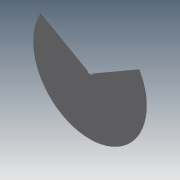
# Autodesk Inventor part: view2
Saved by Autodesk Inventor 2011 (Build 150239000, 239)
## iProperties
Created: 2011-12-04
Part Number: view2
Document SubType Name: Modeling
Designer: Matthew
Density: 1 g/cm^3
Author: Matthew
Autodesk Inventor part; units mm, degrees
ref_plane "YZ Plane" through (0, 0, 0) normal (1, 0, 0) x (0, 1, 0)
ref_plane "XZ Plane" through (0, 0, 0) normal (0, 1, 0) x (-1, 0, 0)
ref_plane "XY Plane" through (0, 0, 0) normal (0, 0, 1) x (1, 0, 0)
sketch "Sketch1" plane through (0, 0, 0) normal (0, 0, 1) x (1, 0, 0)
  arc A0 (-131.9823, 76.2) -> (131.9823, 76.2) centre (0, 0) ccw
  line L0 (6.35, 3.6662) -> (131.9823, 76.2)
  line L1 (0, 0) -> (152.4, 0) construction
  line L2 (-6.35, 3.6662) -> (-85.8668, 49.5752)
  line L3 (0, 0) -> (99.1504, 0) construction
  line L4 (-85.8668, 49.5752) -> (-131.9823, 76.2)
  line L5 (0, 0) -> (6.35, 0)
  line L6 (6.35, 0) -> (6.35, 3.6662)
  line L7 (0, 0) -> (-6.35, 0)
  line L8 (-6.35, 0) -> (-6.35, 3.6662)
  dimension "d0" = 304.8
  dimension "d1" = 30
  dimension "d2" = 150
  dimension "d3" = 6.35
  dimension "d4" = 6.35
  constraints: 18 end point, 3 perpendicular, 2 horizontal, 2 point on circle, 1 centre point, 1 coincident, 1 collinear, 1 point on line
  measures "d0" diameter of A0
  measures "d1" angle of L1 L0
  measures "d2" angle of L3 L2
  measures "d3" distance of L1.start L5.end
  measures "d4" distance of L1.start L7.end
extrude "Extrusion1" add sketch "Sketch1" along normal blind 1
body "Solid1"
